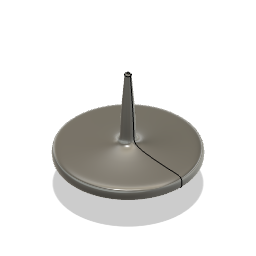
20BL Top v5 (Autodesk Fusion 360 design; units mm, degrees)
Autodesk Fusion 360 part; units mm, degrees
sketch "Top Revolve Profile" plane through (0, 0, 0) normal (0, 0, 1) x (1, 0, 0) in component "5 Min Top"
  spline S0 degree 5 poles (0, 0) (0.0372, 0.0531) (0.1079, 0.157) (0.2026, 0.3064) (0.3063, 0.4924) (0.4006, 0.703) (0.4663, 0.892) (0.5169, 1.06) (0.5757, 1.208) (0.675, 1.3375) (0.8457, 1.45) (1.1101, 1.5466) (1.4716, 1.6273) (1.9122, 1.6915) (2.4011, 1.7387) (2.8998, 1.7695) (3.3683, 1.786) (3.7712, 1.7933) (4.0837, 1.7996) (4.2983, 1.818) (4.4281, 1.8654) (4.4961, 1.9548) (4.5268, 2.089) (4.5357, 2.2514) (4.5273, 2.4128) (4.4961, 2.5444) (4.4269, 2.6309) (4.2962, 2.6772) (4.0827, 2.6981) (3.7741, 2.7115) (3.3773, 2.7289) (2.9155, 2.7557) (2.4217, 2.7936) (1.9336, 2.8416) (1.4884, 2.8982) (1.117, 2.9632) (0.8388, 3.0389) (0.6554, 3.1326) (0.5512, 3.2558) (0.5027, 3.4199) (0.4845, 3.634) (0.4775, 3.9005) (0.4706, 4.2155) (0.4577, 4.5709) (0.4375, 4.9556) (0.411, 5.3579) (0.3806, 5.7662) (0.3486, 6.1718) (0.3163, 6.5683) (0.2849, 6.9517) (0.2547, 7.3195) (0.232, 7.6003) (0.2157, 7.8032) (0.2052, 7.935) (0.2, 8) knots 0 0 0 0 0 0 0.02 0.04 0.06 0.08 0.1 0.12 0.14 0.16 0.18 0.2 0.22 0.24 0.26 0.28 0.3 0.32 0.34 0.36 0.38 0.4 0.42 0.44 0.46 0.48 0.5 0.52 0.54 0.56 0.58 0.6 0.62 0.64 0.66 0.68 0.7 0.72 0.74 0.76 0.78 0.8 0.82 0.84 0.86 0.88 0.9 0.92 0.94 0.96 0.98 1 1 1 1 1 1
  line L0 (0.2, 8) -> (0, 8)
  line L1 (0, 8) -> (0, 0)
  point P0 (0.5, 1)
  point P1 (1, 1.5)
  point P2 (4, 1.8)
  point P3 (4.5, 2)
  point P4 (4.5, 2.5)
  point P5 (4, 2.7)
  point P6 (1, 3)
  point P7 (0.5, 3.5)
  point P8 (0.4, 5.5)
  constraint horizontal L0
  constraint perpendicular L0 L1
revolve "Revolve1" add sketch "Top Revolve Profile" angle 360 about axis through (0, 8, 0) along (0, -1, 0) in component "5 Min Top"
fillet "Fillet1" radius 0.125 1 edges at (-0.1865, 8, -0.0723) in component "5 Min Top"
sketch "Sketch1" plane through (0, 0, 0) normal (0, 0, 1) x (1, 0, 0) in component "Component"
  line L0 (0, 0) -> (22.5, 0) construction
  line L1 (22.5, 0) -> (-22.5, 0) construction
  line L2 (-22.5, 0) -> (-22.5, 35) construction
  line L3 (-22.5, 35) -> (22.5, 35) construction
  line L4 (22.5, 35) -> (22.5, 0) construction
  dimension "d7" = 22.5
  dimension "d8" = 45
  dimension "d9" = 35
  constraint coincident L0.start origin
  constraint horizontal L0
  constraint horizontal L1
  constraint vertical L2
  constraint horizontal L3
  constraint vertical L4
  measures "d7" distance of L0.start L0.end
  measures "d8" distance of L0.end L1.end
  measures "d9" distance of L0.end L3.end
component "5 Min Top" placed x (1, 0, 0) y (0, 1, 0) z (0, 0, 1) at (0, 0, 0)
component "Component" placed x (1, 0, 0) y (0, 1, 0) z (0, 0, 1) at (0, 0, 0)
equation "TopWidth = 45 mm"
equation "TopHeight = 35 mm"
equation "StemWidth = 2.5 mm"
equation "d7 = TopWidth / 2"
equation "d8 = TopWidth"
equation "d9 = TopHeight"
equation "DiskHeight = 5 mm"
named bodies: "Top"
